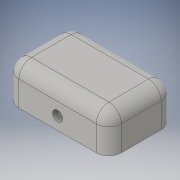
# Autodesk Inventor part: PostCap
Saved by Autodesk Inventor 2016 SP1 (Build 200210100, 210)
## iProperties
Created: 2016-03-07
Part Number: PostCap
Material: Generic
Document SubType Name: Modeling
Designer: steele
Density: 1 g/cm^3
Appearance: Default
Author: steele
Autodesk Inventor part; units mm, degrees
ref_plane "YZ Plane" through (0, 0, 0) normal (1, 0, 0) x (0, 1, 0)
ref_plane "XZ Plane" through (0, 0, 0) normal (0, 1, 0) x (-1, 0, 0)
ref_plane "XY Plane" through (0, 0, 0) normal (0, 0, 1) x (1, 0, 0)
sketch "Sketch1" plane through (0, 0, 0) normal (0, 1, 0) x (-1, 0, 0)
  line L0 (19.558, 10.033) -> (-19.558, 10.033)
  line L1 (-19.558, 10.033) -> (-19.558, -10.033)
  line L2 (-19.558, -10.033) -> (19.558, -10.033)
  line L3 (19.558, -10.033) -> (19.558, 10.033)
  line L4 (19.558, 10.033) -> (-19.558, -10.033) construction
  line L5 (-19.558, 10.033) -> (19.558, -10.033) construction
  line L6 (25.908, 16.383) -> (-25.908, 16.383)
  line L7 (-25.908, 16.383) -> (-25.908, -16.383)
  line L8 (-25.908, -16.383) -> (25.908, -16.383)
  line L9 (25.908, -16.383) -> (25.908, 16.383)
  line L10 (25.908, 16.383) -> (-25.908, -16.383) construction
  line L11 (-25.908, 16.383) -> (25.908, -16.383) construction
  point P0 (0, 0)
  dimension "d0" = 20.066
  dimension "d1" = 39.116
  dimension "d2" = 6.35
  dimension "d3" = 6.35
  constraints: 24 end point, 4 midpoint, 4 parallel, 2 horizontal, 2 perpendicular
  measures "d0" distance of L2.end L0.start
  measures "d1" distance of L0.start L0.end
  measures "d2" distance between parallel lines of L7 L1
  measures "d3" distance between parallel lines of L6 L0
extrude "Extrusion1" add sketch "Sketch1" against normal blind 12.7
sketch "Sketch2" plane through (0, 0, 0) normal (0, 1, 0) x (1, 0, 0)
  line L0 (25.908, -16.383) -> (-25.908, -16.383) projected
  line L1 (-25.908, 16.383) -> (25.908, 16.383) projected
  line L2 (-25.908, -16.383) -> (25.908, -16.383)
  line L3 (25.908, -16.383) -> (25.908, 16.383)
  line L4 (25.908, 16.383) -> (-25.908, 16.383)
  line L5 (-25.908, 16.383) -> (-25.908, -16.383)
  point P0 (0, 0)
  constraints: 8 end point, 2 parallel, 1 horizontal, 1 perpendicular
extrude "Extrusion2" add sketch "Sketch2" along normal blind 6.35
fillet "Fillet1" radius 6.35 4 edges at (0, 6.35, 16.383) (25.908, 6.35, 0) (0, 6.35, -16.383) (-25.908, 6.35, 0)
fillet "Fillet2" radius 6.35 8 edges at (24.0481, 4.4901, 14.5231) (25.908, -6.35, 16.383) (24.0481, 4.4901, -14.5231) (25.908, -6.35, -16.383) (-24.0481, 4.4901, 14.5231) (-25.908, -6.35, 16.383) (-24.0481, 4.4901, -14.5231) (-25.908, -6.35, -16.383)
sketch "Sketch3" plane through (-19.558, -12.7, 16.383) normal (0, 0, 1) x (1, 0, 0)
  line L0 (0, 0) -> (-6.35, 0) construction
  line L1 (45.466, 12.7) -> (39.116, 12.7) construction
  line L2 (0, 0) -> (39.116, 12.7) construction
  line L3 (39.116, 12.7) -> (39.116, 0) construction
  line L4 (0, 19.05) -> (0, 12.7) construction
  line L5 (39.116, 0) -> (0, 12.7) construction
  point P0 (19.558, 12.7)
  point P1 (19.558, 6.35)
  constraints: 4 end point, 1 midpoint
hole "Hole1" at (0, -6.35, 16.383) direction (0, 0, -1) diameter 5.1054 end through all clearance for "Hex Machine Screw" size "#10" standard "Ansi Unified Screw Threads"
equation "\"d0\" = width + 2 * printerError"
equation "\"d1\" = length + 2 * printerError"
equation "\"d2\" = wallThickness"
equation "\"d3\" = wallThickness"
equation "\"d4\" = heightFromTop"
equation "\"d6\" = thicknessAboveTopOfPost"
equation "\"width\" = 19.05"
equation "\"length\" = 38.1"
equation "\"heightFromTop\" = 12.7"
equation "\"thicknessAboveTopOfPost\" = 6.35"
equation "\"printerError\" = 0.508"
equation "\"wallThickness\" = 6.35"
body "Solid1"
